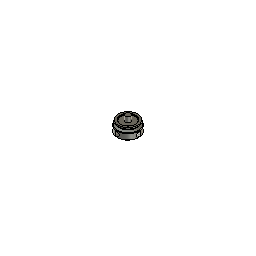
CutterHead_VGroove (Autodesk Fusion 360 design; units mm, degrees)
description: .125" cutters MF104ZZ bearings 2mm belt
Autodesk Fusion 360 part; units mm, degrees
sketch "Sketch1" plane through (0, 0, 0) normal (0, 1, 0) x (1, 0, 0)
  line L0 (0, 6.7947) -> (0, -9.0975)
  line L1 (2, -9.0975) -> (0, -9.0975)
  line L2 (2, -4.8975) -> (2, -9.0975)
  line L3 (7.621, -5.6475) -> (6.05, -5.6475)
  line L4 (7.7395, -4.9005) -> (6.35, -4.4484)
  line L5 (8.495, -2.4737) -> (6.35, -3.1716)
  circle A0 centre (7.62, -3.81) radius 1 construction
  line L6 (8.495, 2.5407) -> (2, 2.5407)
  line L7 (8.495, 2.5407) -> (8.495, -2.4737)
  line L8 (2, 6.7947) -> (2, 2.5407)
  line L9 (2, 6.7947) -> (0, 6.7947)
  circle A1 centre (0, 0) radius 1.7272
  circle A2 centre (0, 0) radius 2.0828 construction
  circle A3 centre (0, 0) radius 1.5875
  line L10 (6.35, -4.4484) -> (6.35, -3.1716)
  arc A4 (7.621, -5.6475) -> (7.7395, -4.9005) centre (7.621, -5.2646) ccw
  circle A5 centre (0, 0) radius 12.7 construction
  circle A6 centre (0, 0) radius 11.1125 construction
  line L11 (5.8, -5.3975) -> (5.8, -5.1475)
  line L12 (5.55, -4.8975) -> (2, -4.8975)
  arc A7 (5.8, -5.3975) -> (6.05, -5.6475) centre (6.05, -5.3975) ccw
  arc A8 (5.8, -5.1475) -> (5.55, -4.8975) centre (5.55, -5.1475) ccw
  line L13 (8.495, -2.4737) -> (0, -2.4737) construction
  dimension "d30" = 2
  dimension "d50" = 0
  dimension "d51" = 0
  dimension "d52" = 0
  dimension "d53" = 0
  dimension "d62" = 0
  dimension "d63" = 0
  dimension "d64" = 0
  dimension "d65" = 0
  dimension "d93" = 3.4544
  dimension "d94" = 4.1656
  dimension "d96" = 3.175
  dimension "d98" = 6.7947
  dimension "d99" = 2
  dimension "d101" = 2
  dimension "d102" = 8.495
  dimension "d110" = 3.81
  dimension "d111" = 7.62
  dimension "d114" = 6.35
  dimension "d116" = 108.025
  dimension "d117" = 108.025
  dimension "d121" = 5.0144
  dimension "d122" = 0.3829
  dimension "d153" = 25.4
  dimension "d154" = 22.225
  dimension "d168" = 5.8
  dimension "d170" = 0.75
  dimension "d175" = 0.25
  dimension "d180" = 0
  dimension "d181" = 0
  dimension "d182" = 0
  dimension "d183" = 0
  dimension "d224" = 4.2
  dimension "d227" = 15.8922
  constraint tangent L4 A0
  constraint tangent L5 A0
  constraint vertical L8
  constraint perpendicular L0 L9
  constraint coincident A1.centre A2.centre
  constraint vertical L0
  constraint horizontal L1
  constraint vertical L10
  constraint tangent L4 A4
  constraint tangent L3 A4
  constraint horizontal L3
  constraint vertical L2
  constraint vertical L7
  constraint concentric A1 A5
  constraint concentric A3 A6
  constraint perpendicular L3 L11
  constraint perpendicular L11 L12
  constraint tangent L11 A7
  constraint tangent L3 A7
  constraint tangent L11 A8
  constraint tangent L12 A8
  constraint equal A7 A8
  constraint coincident L0 L13.end
  constraint perpendicular L0 L13
  constraint horizontal L6
  constraint coincident L0 A1.centre
  measures "d30" diameter of A0
  measures "d93" diameter of A1
  measures "d94" diameter of A2
  measures "d96" diameter of A3
  measures "d98" distance of L9 A1.centre
  measures "d99" distance of L8.start L0.start
  measures "d101" distance of L0.end L1.start
  measures "d102" distance of A1.centre L7
  measures "d110" vertical distance of A0.centre A1.centre
  measures "d111" horizontal distance of A0.centre A1.centre
  measures "d114" distance of A1.centre L10
  measures "d116" angle of L5 L10
  measures "d117" angle of L4 L10
  measures "d121" distance of L6.start L5.start
  measures "d153" diameter of A5
  measures "d154" diameter of A6
  measures "d168" distance of A1.centre L11
  measures "d170" distance of L3 L12
  measures "d175" radius of A7
  measures "d224" distance of L1.start L2.start
  measures "d227" distance of L0.end L0.start
revolve "Revolve3" add sketch "Sketch1" angle 360 about axis through (0, 0, -6.7947) along (0, 0, 1) contours L0 L1 L2 L3 L4 L5 L6 L7 L8 L9 A1 L10 A4 L11 L12 A7 A8 | L0 A1 A3 | L0 A3 picked at (0.0819, -1.6748) picked at (0.3465, 0.3999)
extrude "Extrude5" cut sketch "Sketch1" along normal mid plane 28.2346 contours L0 A1 A3 | L0 A1 A3 | L0 A3 | L0 A3
move_face "MoveFace2" to x (0, 1, 0) y (-1, 0, 0) z (0, 0, 1) at (0.0002, -0.0002, 0) 1 faces at (0.425, -2.8249, -1.6741)
extrude "Extrude6" cut sketch "Sketch1" along normal mid plane 24.5974 contours L0 A3 | L0 A3
thread "Thread2" "ANSI Unified Screw Threads 0.164(#8) 8-32 UNC 3B" major diameter 4.1656 minor diameter 3.4163 pitch 0.7937 angle 60 resizes the face on face at (0.008, -0.4552, 1.6662)
fillet "Fillet2" radius 0.508 2 edges at (-7.9201, -3.0719, 2.4737) (-7.9201, -3.0719, -2.5407)
equation "d101 = d99"
equation "d117 = d116"
equation "d168 = ( 11.6 / 2 ) * 1 mm"
